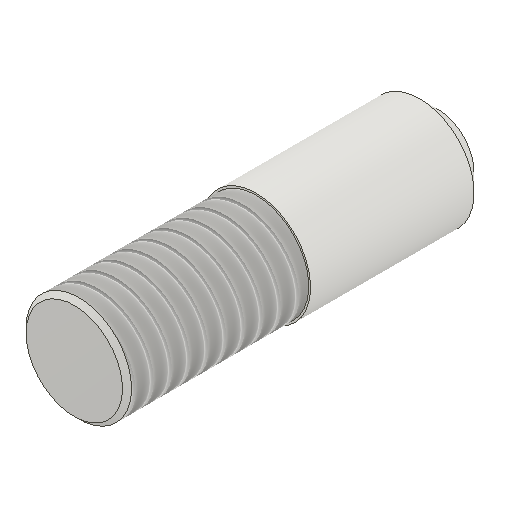
# Autodesk Inventor part: GRJ-03-118
Saved by Autodesk Inventor 2026.1 (Build 301233000, 233)
## iProperties
Company: Gree
Created: 2025-08-20
Part Number: GRJ-03-118
Checked By: Antonio Lucas
Engr Approved By: Antonio Lucas
Material: Aço SAE 1045
Document SubType Name: Modeling
Mfg Approved By: Anderson Oliveira
Designer: Willian Pinheiro
Mass: 4.22346 g
Surface Area: 4.12164 cm^2
Volume: 0.538021 cm^3
Density: 7.85 g/cm^3
Appearance: Aço
Description: Eixo Roscado Ø6
Project: GRJ-03
Dimensões: Ø6 x 20 mm
Total: 1
Author: Willian Pinheiro
Revision Number: 00
Title: Soldagem
Autodesk Inventor part; units mm, degrees
ref_plane "YZ Plane" through (0, 0, 0) normal (1, 0, 0) x (0, 1, 0)
ref_plane "XZ Plane" through (0, 0, 0) normal (0, 1, 0) x (-1, 0, 0)
ref_plane "XY Plane" through (0, 0, 0) normal (0, 0, 1) x (1, 0, 0)
sketch "Esboço1" plane through (0, 0, 0) normal (0, 0, 1) x (1, 0, 0)
  line L0 (-3.6, 0) -> (0.6, 0) construction
  line L1 (0, -14) -> (0, 14) construction
  line L2 (-3, 10) -> (0, 10)
  line L3 (0, 10) -> (0, -10)
  line L4 (0, -10) -> (-3, -10)
  line L5 (-3, -10) -> (-3, 10)
  line L6 (-3, 0) -> (-2.9, 0)
  line L7 (-2.9, 0) -> (-2.9, -10)
  line L8 (-2, 10) -> (-3, 9)
  line L9 (-2.9, -9.75) -> (-2.65, -10)
  line L10 (-3, 0.25) -> (-2.9, 0.15)
  point P0 (0, 0)
  point P1 (-2.75, 0)
  dimension "d0" = 6
  dimension "d1" = 5.8
  dimension "d2" = 10
  dimension "d3" = 20
  dimension "d4" = 1
  dimension "d5" = 1
  dimension "d6" = 0.25
  dimension "d7" = 0.25
  dimension "d8" = 45
  dimension "d12" = 0.25
  constraints: 18 end point, 8 point on line, 2 horizontal, 2 parallel, 2 perpendicular, 1 midpoint, 1 other
  measures "d0" diameter of L5 L3
  measures "d1" diameter of L7 L3
  measures "d2" distance between parallel lines of L2 L6
  measures "d3" distance between parallel lines of L4 L2
  measures "d4" horizontal distance of L8.start L8.end
  measures "d5" horizontal distance of L8.start L8.end
  measures "d6" horizontal distance of L9.start L9.end
  measures "d7" horizontal distance of L9.start L9.end
  measures "d8" angle of L6 L10
  measures "d12" distance from line of L0 L10.start
revolve "Revolução1" add sketch "Esboço1" angle 360 about axis through (0, 10, 0) along (0, -1, 0) contours L2 L3 L4 L9 L7 L6 L5 L8
thread "Rosca1" size "M6x1" class "6g" standard "ISO Metric profile" full length
equation "\"d6\" = d7"
